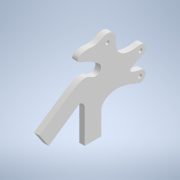
# Autodesk Inventor part: lamina_eje_trasero
Saved by Autodesk Inventor 2021 (Build 250183000, 183)
## iProperties
Created: 2021-04-09
Part Number: lamina_eje_trasero
Material: Genérico
Document SubType Name: Modeling
Designer: j2seb
Density: 1 g/cm^3
Appearance: Valor por defecto
Author: j2seb
Autodesk Inventor part; units mm, degrees
ref_plane "YZ Plane" through (0, 0, 0) normal (1, 0, 0) x (0, 1, 0)
ref_plane "XZ Plane" through (0, 0, 0) normal (0, 1, 0) x (-1, 0, 0)
ref_plane "XY Plane" through (0, 0, 0) normal (0, 0, 1) x (1, 0, 0)
sketch "Boceto1" plane through (0, 0, 0) normal (1, 0, 0) x (0, 1, 0)
  line L0 (-20.1912, -7.3118) -> (-34.868, -7.3118) construction
  spline S0 degree 4 poles (-29.6871, -38.5039) (-24.1556, -26.0638) (-21.7281, -18) (-20.1912, -7.3118) (-34.868, -7.3118) knots 21.570729 21.570729 21.570729 21.570729 21.570729 22 22 22 22 22
  line L1 (-29.6871, -38.5039) -> (-24.1556, -26.0638) construction
  line L2 (-24.1556, -26.0638) -> (-21.7281, -18) construction
  line L3 (-21.7281, -18) -> (-20.1912, -7.3118) construction
  line L4 (-50, 13.9603) -> (0, 0) construction
  line L5 (0, 0) -> (-50, 0) construction
  arc A0 (-29.6871, -38.5039) -> (-20.1912, -41.3852) centre (-25.1184, -40.5354) ccw
  line L6 (-16.7423, -21.3881) -> (-20.1912, -41.3852) construction
  spline S1 degree 2 poles (-9.815, -42.481) (-16.7423, -21.3881) (-20.1912, -41.3852) knots 1 1 1 2 2 2
  line L7 (-9.815, -42.481) -> (-16.7423, -21.3881) construction
  line L8 (2.3245, 8.0391) -> (-2.902, 7.319) construction
  spline S2 degree 4 poles (-18.9531, 38.3459) (-1.6814, 14.9192) (2.3245, 8.0391) (-2.902, 7.319) (-4.5878, 1.2809) knots 1 1 1 1 1 2 2 2 2 2
  line L9 (-18.9531, 38.3459) -> (-1.6814, 14.9192) construction
  line L10 (-1.6814, 14.9192) -> (2.3245, 8.0391) construction
  line L11 (-2.902, 7.319) -> (-4.5878, 1.2809) construction
  line L12 (3.7767, -2.9026) -> (9.4181, 4.4375) construction
  spline S3 degree 4 poles (3.7767, -2.9026) (9.4181, 4.4375) (12.4291, 11.3201) (14.6356, 22.4473) (23.4504, 7.8788) (17.807, 0.7674) (21.8821, -3.919) (23.3738, -8.5503) knots 0 0 0 0 0 1 2 3 4 4 4 4 4
  line L13 (9.4181, 4.4375) -> (12.4291, 11.3201) construction
  line L14 (12.4291, 11.3201) -> (14.6356, 22.4473) construction
  line L15 (14.6356, 22.4473) -> (23.4504, 7.8788) construction
  line L16 (23.4504, 7.8788) -> (17.807, 0.7674) construction
  line L17 (17.807, 0.7674) -> (21.8821, -3.919) construction
  line L18 (21.8821, -3.919) -> (23.3738, -8.5503) construction
  circle A1 centre (0, 0) radius 4.7633
  arc A2 (15.9103, -18.3426) -> (23.3738, -8.5503) centre (16.2349, -10.8497) ccw
  line L19 (-34.0809, 46.2261) -> (0, 0) construction
  arc A3 (-9.815, -42.481) -> (-0.1292, -40.1199) centre (-5.0647, -40.9208) ccw
  line L20 (-3.5244, -19.1976) -> (-0.1292, -40.1199) construction
  spline S4 degree 3 poles (15.9103, -18.3426) (8, -18) (-3.5244, -19.1976) (-0.1292, -40.1199) knots 1 1 1 1 2 2 2 2
  line L21 (15.9103, -18.3426) -> (8, -18) construction
  line L22 (8, -18) -> (-3.5244, -19.1976) construction
  line L23 (-31.0868, 29.5264) -> (-40.1176, 41.7755)
  line L24 (-28.0441, 50.6768) -> (-18.9531, 38.3459)
  line L25 (-40.1176, 41.7755) -> (-28.0441, 50.6768)
  line L26 (-34.868, -7.3118) -> (-54.868, -7.3118)
  line L27 (-54.868, -7.3118) -> (-54.868, 7.6882)
  line L28 (-54.868, 7.6882) -> (-25, 7.6882)
  line L29 (-25, 7.6882) -> (-24.868, 7.6882)
  arc A4 (-24.868, 7.6882) -> (-17.9191, 11.6663) centre (-24.868, 15.7464) ccw
  line L30 (-17.9191, 11.6663) -> (-31.0868, 29.5264)
  point P0 (3.7768, -2.9026)
  dimension "d1" = 38
  dimension "d3" = 9.5266
  dimension "d4" = 15
  dimension "d5" = 10
  dimension "d6" = 10
  dimension "d7" = 344.4
  dimension "d25" = 20
  dimension "d26" = 15
  dimension "d28" = 15
  dimension "d29" = 30
  dimension "d30" = 30
  constraints: 22 end point, 10 point on circle, 5 centre point, 5 coincident, 3 horizontal, 3 perpendicular, 2 parallel, 2 point on line, 1 collinear, 1 midpoint, 1 tangent, 24 other
  measures "d1" angle of L4 L19
  measures "d3" diameter of A1
  measures "d4" diameter of A2
  measures "d5" diameter of A3
  measures "d6" diameter of A0
  measures "d25" distance of L0.end L26.end
  measures "d26" distance of L26.end L27.end
  measures "d28" distance between parallel lines of L23 L24
  measures "d29" distance from line of A4.centre L25
  measures "d30" distance from line of L27 A4.centre
extrude "Extrusión1" add sketch "Boceto1" along normal mid plane 5 contours S0 L26 L27 L28 L29 A4 L30 L23 L25 L24 S2 A1 S3 A2 S4 A3 S1 A0
sketch "Boceto2" plane through (2.5, 0, 0) normal (1, 0, 0) x (0, 0, -1)
  arc A0 (18.3426, 15.9103) -> (8.5503, 23.3738) centre (10.8497, 16.2349) ccw projected
  point P0 (0, 0)
  constraints: 1 coincident
hole "Agujero1" at (2.5, 16.2349, -10.8497) direction (-1, 0, 0) diameter 3.4 end through all clearance for "Tornillo para maquinaria de cabeza plana" size "M3" standard "Perfil M métrico ANSI"
sketch "Boceto3" plane through (2.5, 0, 0) normal (1, 0, 0) x (0, 0, -1)
  arc A0 (42.481, -9.815) -> (40.1199, -0.1292) centre (40.9208, -5.0647) ccw projected
  arc A1 (38.5039, -29.6871) -> (41.3852, -20.1912) centre (40.5354, -25.1184) ccw projected
  point P0 (0, 0)
  constraints: 2 coincident
hole "Agujero2" at (2.5, -5.0647, -40.9208) at (2.5, -25.1184, -40.5354) direction (-1, 0, 0) diameter 3.4 end through all clearance for "Tornillo para maquinaria de cabeza plana" size "M3" standard "Perfil M métrico ANSI"
